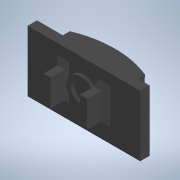
# Autodesk Inventor part: Finger Button
Saved by Autodesk Inventor 2020 (Build 240168000, 168)
## iProperties
Created: 2021-05-05
Part Number: Finger Button
Material: Generic
Document SubType Name: Modeling
Designer: Luke
Density: 1 g/cm^3
Appearance: Default
Author: Luke
Autodesk Inventor part; units mm, degrees
ref_plane "YZ Plane" through (0, 0, 0) normal (1, 0, 0) x (0, 1, 0)
ref_plane "XZ Plane" through (0, 0, 0) normal (0, 1, 0) x (-1, 0, 0)
ref_plane "XY Plane" through (0, 0, 0) normal (0, 0, 1) x (1, 0, 0)
sketch "Sketch1" plane through (0, 0, 0) normal (0, 1, 0) x (-1, 0, 0)
  line L0 (0, 0) -> (-16, 0)
  line L1 (-16, 0) -> (-16, -5)
  line L2 (0, -5) -> (0, 0)
  arc A0 (-16, -5) -> (0, -5) centre (-8, 14.291) ccw
  dimension "d0" = 16
  dimension "d1" = 5
  constraints: 6 end point, 2 point on circle, 1 centre point, 1 horizontal, 1 parallel, 1 perpendicular
  measures "d0" distance of L2.start L1.end
  measures "d1" distance of L1.end L0.end
extrude "Extrusion1" add sketch "Sketch1" along normal blind 13
sketch "Sketch2" plane through (0, 0, 0) normal (0, 0, 1) x (1, 0, 0)
  line L0 (16, 13) -> (0, 13) projected
  line L1 (0, 13) -> (0.6813, 0)
  line L2 (16, 0) -> (0, 0) projected
  line L3 (0, 13) -> (13.0178, 13) construction
  line L4 (0.6813, 0) -> (0, 0)
  line L5 (0, 0) -> (0, 13) projected
  line L6 (0, 0) -> (0, 13)
  line L7 (16, 13) -> (15.3187, 0)
  line L8 (16, 13) -> (29.0178, 13) construction
  line L9 (15.3187, 0) -> (16, 0)
  line L10 (16, 0) -> (16, 13) projected
  line L11 (16, 13) -> (16, 0)
  dimension "d4" = 87
  dimension "d5" = 93
  constraints: 16 end point, 2 collinear, 2 equal length, 2 horizontal, 2 point on line, 1 perpendicular
  measures "d4" angle of L1 L3
  measures "d5" angle of L7 L8
extrude "Extrusion2" cut sketch "Sketch2" against normal through all contours L10 L2 L7 | L1 L2 L5
sketch "Sketch3" plane through (0.6813, 0, 0) normal (0, 0, 1) x (1, 0, 0)
  line L0 (7.3187, 0) -> (7.3187, -1.8081)
  line L1 (-4.6813, 13) -> (-4.6813, 14.5)
  line L2 (19.3187, 0) -> (19.3187, -1.5)
  line L3 (-4.6813, 14.5) -> (19.3187, 14.5)
  line L4 (19.3187, 14.5) -> (19.3187, -1.5)
  line L5 (19.3187, -1.5) -> (-4.6813, -1.5)
  line L6 (-4.6813, -1.5) -> (-4.6813, 14.5)
  point P0 (-4.6813, 0)
  point P1 (19.3187, 13)
  point P2 (19.3187, 0)
  dimension "d17" = 1.5
  dimension "d18" = 1.5
  constraints: 14 end point, 3 vertical, 2 parallel, 1 horizontal, 1 perpendicular
  measures "d17" distance of L1.start L1.end
  measures "d18" distance of L2.start L2.end
extrude "Extrusion3" add sketch "Sketch3" against normal blind 2
sketch "Sketch5" plane through (-4, -1.5, 0) normal (0, 0, 1) x (1, 0, 0)
  line L0 (24, 16) -> (0, 16) projected
  line L1 (12, 16) -> (12, 10)
  line L2 (12, 16) -> (18, 16) construction
  circle A0 centre (12, 10) radius 2
  circle A1 centre (12, 10) radius 3
  point P0 (4, 1.5)
  dimension "d21" = 6
  dimension "d22" = 90
  dimension "d23" = 4
  dimension "d24" = 1
  constraints: 4 end point, 2 centre point, 2 perpendicular, 1 coincident, 1 horizontal, 1 midpoint
  measures "d21" distance of L1.start L1.end
  measures "d22" angle of L1 L2
  measures "d23" diameter of A0
  measures "d24" radial gap between concentric circles of A0 A1
extrude "Extrusion5" add sketch "Sketch5" along normal blind 0.7
ref_plane "Work Plane1" through (8, -1.5, 0) normal (1, 0, 0) x (0, 0, -1)
sketch "Sketch7" plane through (-4, -1.5, 0) normal (0, 0, 1) x (1, 0, 0)
  circle A0 centre (12, 10) radius 1.8
  line L0 (15.1, 12.85) -> (15.1, 7.15)
  line L1 (12, 10) -> (12, 10.6806)
  line L2 (15.1, 7.15) -> (15.15, 7.15)
  line L3 (15.15, 7.15) -> (16.65, 7.15)
  line L4 (16.65, 7.15) -> (16.65, 12.85)
  line L5 (16.65, 12.85) -> (15.15, 12.85)
  line L6 (15.15, 12.85) -> (15.15, 7.15)
  line L7 (8.85, 7.15) -> (7.35, 7.15)
  line L8 (7.35, 7.15) -> (7.35, 12.85)
  line L9 (7.35, 12.85) -> (8.85, 12.85)
  line L10 (8.85, 12.85) -> (8.85, 7.15)
  point P0 (4, 1.5)
  dimension "d59" = 0.05
  dimension "d60" = 1.5
  constraints: 22 end point, 4 symmetric about line, 2 horizontal, 2 parallel, 1 centre point, 1 coincident, 1 perpendicular, 1 vertical
  measures "d59" distance of L0.end L2.end
  measures "d60" distance of L5.end L4.end
extrude "Extrusion6" add sketch "Sketch7" along normal blind 4 contours L6 L5 L4 L3 | L7 L8 L9 L10
sketch "Sketch8" plane through (-4, -1.5, 0) normal (-1, 0, 0) x (0, 0, 1)
  line L0 (0.479, 3) -> (-2, 3)
  line L1 (-2, 4.5) -> (-5.2686, 4.5)
  line L2 (-5.2686, 4.5) -> (-7, 4.5)
  line L3 (-5.2686, 4.5) -> (-3.5373, 4.5) construction
  line L4 (-7, 4.5) -> (-7, -1.1615)
  line L5 (-7, -1.1615) -> (0.479, -1.1615)
  line L6 (0.479, -1.1615) -> (0.479, 3)
  line L7 (-2, 3) -> (-2, 4.5)
  dimension "d48" = 180
  constraints: 16 end point, 2 perpendicular, 1 collinear, 1 horizontal, 1 vertical
  measures "d48" angle of L2 L3
extrude "Extrusion7" cut sketch "Sketch8" against normal through all
chamfer "Chamfer2" distance 1 angle 45 6 edges at (4.1, 11.35, 0) (3.35, 8.5, 0) (4.1, 5.65, 0) (11.9, 11.35, 0) (12.65, 8.5, 0) (11.9, 5.65, 0)
chamfer "Chamfer3" distance 0.2 angle 45 1 edges at (6, 8.5, 0.7)
body "Solid1"
